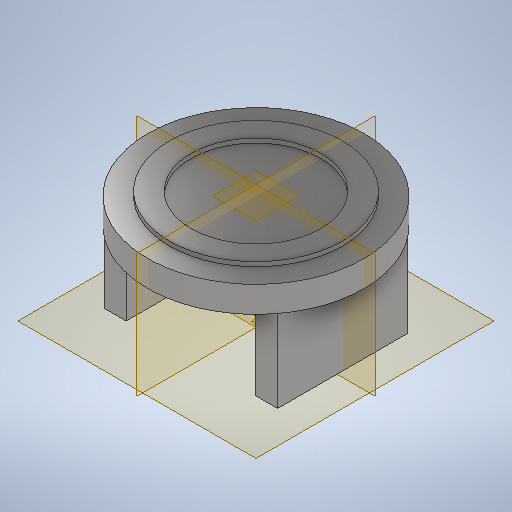
# Autodesk Inventor part: Z5
Saved by Autodesk Inventor 2025.2 (Build 292293000, 293)
## iProperties
Created: 2025-03-23
Part Number: Z5
Material: Steel, Alloy
Document SubType Name: Modeling
Designer: MSIGAMING
Density: 7.73 g/cm^3
Appearance: Semi-Polished
Mass: 1247.99 g
Surface Area: 301.179 cm^2
Volume: 161.448 cm^3
Author: MSIGAMING
Autodesk Inventor part; units mm, degrees
ref_plane "Work Plane1" through (0, 50, 0) normal (0, 1, 0) x (-1, 0, 0)
sketch "Sketch1" plane through (0, 50, 0) normal (0, 1, 0) x (-1, 0, 0)
  circle A0 centre (0, 0) radius 50
  dimension "d11" = 100
  constraints: 1 centre point
  measures "d11" diameter of A0
extrude "Extrusion1" add sketch "Sketch1" against normal blind 12
sketch "Sketch2" plane through (0, 0, 0) normal (0, 0, 1) x (1, 0, 0)
  line L0 (-40, 38) -> (40, 38) projected
  line L1 (-40, 50) -> (-40, 38) projected
  line L2 (-40, 38) -> (-40, 0)
  line L3 (-40, 0) -> (-30, 0)
  line L4 (-30, 0) -> (-30, 32)
  line L5 (-30, 32) -> (30, 32)
  line L6 (30, 32) -> (30, 0)
  line L7 (30, 0) -> (40, 0)
  line L8 (40, 50) -> (40, 38) projected
  line L9 (40, 0) -> (40, 38)
  point P0 (0, 0)
  dimension "d5" = 10
  dimension "d6" = 32
  dimension "d7" = 60
  dimension "d8" = 10
  constraints: 14 end point, 3 perpendicular, 2 point on line, 1 parallel, 1 vertical
  measures "d5" distance of L2.end L3.end
  measures "d6" distance of L3.end L4.end
  measures "d7" distance of L4.end L5.end
  measures "d8" distance of L6.end L7.end
extrude "Extrusion2" add sketch "Sketch2" along normal mid plane 60
sketch "Sketch3" plane through (0, 50, 0) normal (0, 1, 0) x (1, 0, 0)
  circle A0 centre (0, 0) radius 40
  circle A1 centre (0, 0) radius 30
  dimension "d12" = 80
  dimension "d15" = 60
  constraints: 2 centre point, 2 coincident
  measures "d12" diameter of A0
  measures "d15" diameter of A1
extrude "Extrusion3" add sketch "Sketch3" along normal blind 2
body "Solid1"
